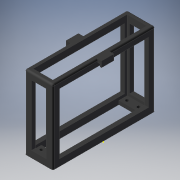
# Autodesk Inventor part: Battery Case2
Saved by Autodesk Inventor 2019 (Build 230136000, 136)
## iProperties
Created: 2019-01-06
Part Number: Battery Case2
Material: Generic
Document SubType Name: Modeling
Designer: Ashley
Density: 1 g/cm^3
Appearance: Default
Author: Ashley
Autodesk Inventor part; units mm, degrees
ref_plane "YZ Plane" through (0, 0, 0) normal (1, 0, 0) x (0, 1, 0)
ref_plane "XZ Plane" through (0, 0, 0) normal (0, 1, 0) x (-1, 0, 0)
ref_plane "XY Plane" through (0, 0, 0) normal (0, 0, 1) x (1, 0, 0)
sketch "Sketch1" plane through (0, 0, 0) normal (0, 1, 0) x (-1, 0, 0)
  point P0 (0, 0)
sketch "Sketch2" plane through (0, 0, 0) normal (0, 1, 0) x (-1, 0, 0)
  line L0 (34.7144, 60.4703) -> (0.7144, 60.4703)
  line L1 (0.7144, 60.4703) -> (0.7144, -63.8297)
  line L2 (0.7144, -63.8297) -> (34.7144, -63.8297)
  line L3 (34.7144, -63.8297) -> (34.7144, 60.4703)
  point P0 (0, 0)
  dimension "d0" = 124.3
  dimension "d1" = 34
  constraints: 8 end point, 2 parallel, 1 horizontal, 1 perpendicular
  measures "d0" distance of L2.end L0.start
  measures "d1" distance of L0.start L0.end
extrude "Extrusion1" add sketch "Sketch2" along normal blind 90
sketch "Sketch3" plane through (0, 90, 0) normal (0, 1, 0) x (1, 0, 0)
  line L0 (-34.7144, -60.4703) -> (-0.7144, -60.4703) construction
  line L1 (-0.7144, -60.4703) -> (-0.7144, 63.8297) construction
  line L2 (-0.7144, 63.8297) -> (-34.7144, 63.8297) construction
  line L3 (-34.7144, 63.8297) -> (-34.7144, -60.4703) construction
  line L4 (-29.7144, 58.8297) -> (-5.7144, 58.8297)
  line L5 (-5.7144, 58.8297) -> (-5.7144, -55.4703)
  line L6 (-5.7144, -55.4703) -> (-29.7144, -55.4703)
  line L7 (-29.7144, -55.4703) -> (-29.7144, 58.8297)
  point P0 (0, 0)
  dimension "d4" = 114.3
  dimension "d5" = 24
  dimension "d6" = 5
  dimension "d7" = 5
  dimension "d8" = 5
  dimension "d9" = 5
  constraints: 8 end point, 2 parallel, 1 horizontal, 1 perpendicular
  measures "d4" distance of L6.end L4.start
  measures "d5" distance of L5.end L6.end
  measures "d6" distance between parallel lines of L1 L5
  measures "d7" distance between parallel lines of L3 L7
  measures "d8" distance between parallel lines of L0 L6
  measures "d9" distance between parallel lines of L2 L4
extrude "Extrusion2" cut sketch "Sketch3" against normal blind 85.5
sketch "Sketch4" plane through (-0.7144, 0, 60.4703) normal (1, 0, 0) x (0, 0, -1)
  line L0 (124.3, 0) -> (124.3, 90) construction
  line L1 (0, 90) -> (124.3, 90) construction
  line L2 (54.65, 90) -> (69.65, 90)
  line L3 (69.65, 90) -> (69.65, 83)
  line L4 (69.65, 83) -> (54.65, 83)
  line L5 (54.65, 83) -> (54.65, 90)
  point P0 (60.4703, 0)
  dimension "d12" = 15
  dimension "d13" = 7
  dimension "d14" = 0
  dimension "d15" = 54.65
  constraints: 8 end point, 2 parallel, 1 horizontal, 1 perpendicular
  measures "d12" distance of L2.start L2.end
  measures "d13" distance of L2.end L3.end
  measures "d14" distance between parallel lines of L1 L2
  measures "d15" distance between parallel lines of L0 L3
extrude "Extrusion3" add sketch "Sketch4" along normal blind 4.5
sketch "Sketch5" plane through (-34.7144, 0, -63.8297) normal (-1, 0, 0) x (0, 0, 1)
  line L0 (124.3, 0) -> (124.3, 90) construction
  line L1 (0, 90) -> (124.3, 90) construction
  line L2 (54.65, 90) -> (69.65, 90)
  line L3 (69.65, 90) -> (69.65, 83)
  line L4 (69.65, 83) -> (54.65, 83)
  line L5 (54.65, 83) -> (54.65, 90)
  point P0 (63.8297, 0)
  dimension "d18" = 7
  dimension "d19" = 15
  dimension "d20" = 0
  dimension "d21" = 54.65
  constraints: 8 end point, 2 parallel, 1 horizontal, 1 perpendicular
  measures "d18" distance of L2.end L3.end
  measures "d19" distance of L3.end L4.end
  measures "d20" distance between parallel lines of L1 L2
  measures "d21" distance between parallel lines of L0 L3
extrude "Extrusion4" add sketch "Sketch5" along normal blind 4.5
sketch "Sketch6" plane through (-34.7144, 83, -9.1797) normal (0, -1, 0) x (1, 0, 0)
  line L0 (0, 15) -> (0, 0) construction
  line L1 (0, 15) -> (-4.5, 15) construction
  line L2 (-3, 0) -> (0, 0)
  line L3 (0, 0) -> (0, 15)
  line L4 (0, 15) -> (-3, 15)
  line L5 (-3, 15) -> (-3, 0)
  point P0 (34.7144, 9.1797)
  dimension "d24" = 15
  dimension "d25" = 3
  dimension "d26" = 0
  dimension "d27" = 0
  constraints: 8 end point, 2 parallel, 1 horizontal, 1 perpendicular
  measures "d24" distance of L4.end L2.start
  measures "d25" distance of L3.end L4.end
  measures "d26" distance between parallel lines of L0 L3
  measures "d27" distance between parallel lines of L1 L4
extrude "Extrusion5" cut sketch "Sketch6" against normal blind 3
sketch "Sketch7" plane through (-0.7144, 83, -9.1797) normal (0, -1, 0) x (1, 0, 0)
  line L0 (0, 0) -> (0, 15) construction
  line L1 (0, 15) -> (4.5, 15) construction
  line L2 (0, 15) -> (3, 15)
  line L3 (3, 15) -> (3, 0)
  line L4 (3, 0) -> (0, 0)
  line L5 (0, 0) -> (0, 15)
  point P0 (0.7144, 9.1797)
  dimension "d30" = 15
  dimension "d31" = 3
  dimension "d32" = 0
  dimension "d33" = 0
  constraints: 8 end point, 2 parallel, 1 horizontal, 1 perpendicular
  measures "d30" distance of L2.end L3.end
  measures "d31" distance of L2.start L2.end
  measures "d32" distance between parallel lines of L1 L2
  measures "d33" distance between parallel lines of L5 L0
extrude "Extrusion6" cut sketch "Sketch7" against normal blind 3
sketch "Sketch8" plane through (-34.7144, 0, 60.4703) normal (0, 0, 1) x (1, 0, 0)
  line L0 (0, 0) -> (34, 0) construction
  line L1 (34, 0) -> (34, 90) construction
  line L2 (0, 90) -> (34, 90) construction
  line L3 (0, 0) -> (0, 90) construction
  line L4 (8, 82) -> (26, 82)
  line L5 (26, 82) -> (26, 8)
  line L6 (26, 8) -> (8, 8)
  line L7 (8, 8) -> (8, 82)
  point P0 (34.7144, 0)
  dimension "d38" = 8
  dimension "d39" = 8
  dimension "d84" = 8
  dimension "d85" = 8
  constraints: 8 end point, 2 parallel, 1 horizontal, 1 perpendicular
  measures "d38" distance between parallel lines of L1 L5
  measures "d39" distance between parallel lines of L2 L4
  measures "d84" distance between parallel lines of L3 L7
  measures "d85" distance between parallel lines of L6 L0
extrude "Extrusion7" cut sketch "Sketch8" against normal blind 124.3
sketch "Sketch9" plane through (-0.7144, 0, 60.4703) normal (1, 0, 0) x (0, 0, -1)
  line L0 (0, 0) -> (0, 90) construction
  line L1 (0, 0) -> (124.3, 0) construction
  line L2 (124.3, 0) -> (124.3, 90) construction
  line L3 (69.65, 90) -> (124.3, 90) construction
  line L4 (8, 82) -> (116.3, 82)
  line L5 (116.3, 82) -> (116.3, 8)
  line L6 (116.3, 8) -> (8, 8)
  line L7 (8, 8) -> (8, 82)
  point P0 (60.4703, 0)
  dimension "d46" = 8
  dimension "d48" = 8
  dimension "d82" = 8
  dimension "d83" = 8
  constraints: 8 end point, 2 parallel, 1 horizontal, 1 perpendicular
  measures "d46" distance between parallel lines of L0 L7
  measures "d48" distance between parallel lines of L3 L4
  measures "d82" distance between parallel lines of L2 L5
  measures "d83" distance between parallel lines of L6 L1
extrude "Extrusion8" cut sketch "Sketch9" against normal blind 34
sketch "Sketch11" plane through (0, 0, 0) normal (0, -1, 0) x (1, 0, 0)
  line L0 (-34.7144, 60.4703) -> (-0.7144, 60.4703) construction
  line L1 (-34.7144, -63.8297) -> (-34.7144, 60.4703) construction
  line L2 (-0.7144, -63.8297) -> (-34.7144, -63.8297) construction
  line L3 (-0.7144, 60.4703) -> (-0.7144, -63.8297) construction
  circle A0 centre (-24.7144, -53.8297) radius 2.1
  circle A1 centre (-10.7144, -53.8297) radius 2.1
  circle A2 centre (-24.7144, 50.4703) radius 2.1
  circle A3 centre (-10.7144, 50.4703) radius 2.1
  line L4 (-29.7144, -48.8297) -> (-5.7144, -48.8297)
  line L5 (-5.7144, -48.8297) -> (-5.7144, 45.4703)
  line L6 (-5.7144, 45.4703) -> (-29.7144, 45.4703)
  line L7 (-29.7144, 45.4703) -> (-29.7144, -48.8297)
  point P0 (0, 0)
  dimension "d52" = 4.2
  dimension "d53" = 10
  dimension "d54" = 10
  dimension "d55" = 4.2
  dimension "d56" = 10
  dimension "d57" = 10
  dimension "d58" = 4.2
  dimension "d59" = 10
  dimension "d60" = 10
  dimension "d61" = 4.2
  dimension "d62" = 10
  dimension "d63" = 10
  dimension "d66" = 94.3
  dimension "d67" = 24
  dimension "d68" = 5
  dimension "d69" = 5
  dimension "d70" = 5
  dimension "d71" = 5
  constraints: 8 end point, 4 centre point, 2 parallel, 1 horizontal, 1 perpendicular
  measures "d52" diameter of A0
  measures "d53" distance from line of L2 A0.centre
  measures "d54" distance from line of L1 A0.centre
  measures "d55" diameter of A1
  measures "d56" distance from line of L2 A1.centre
  measures "d57" distance from line of L3 A1.centre
  measures "d58" diameter of A2
  measures "d59" distance from line of L0 A2.centre
  measures "d60" distance from line of L1 A2.centre
  measures "d61" diameter of A3
  measures "d62" distance from line of L0 A3.centre
  measures "d63" distance from line of L3 A3.centre
  measures "d66" distance of L6.end L4.start
  measures "d67" distance of L5.end L6.end
  measures "d68" distance from line of A2.centre L6
  measures "d69" distance from line of A0.centre L4
  measures "d70" distance between parallel lines of L1 L7
  measures "d71" distance between parallel lines of L3 L5
extrude "Extrusion9" cut sketch "Sketch11" against normal blind 5 contours A0 | A1 | A2 | A3
sketch "Sketch12" plane through (0, 0, 0) normal (0, -1, 0) x (1, 0, 0)
  circle A0 centre (-24.7144, 50.4703) radius 2.1 construction
  circle A1 centre (-24.7144, -53.8297) radius 2.1 construction
  line L0 (-34.7144, -63.8297) -> (-34.7144, 60.4703) construction
  line L1 (-0.7144, 60.4703) -> (-0.7144, -63.8297) construction
  line L2 (-29.7144, -48.8297) -> (-5.7144, -48.8297)
  line L3 (-5.7144, -48.8297) -> (-5.7144, 45.4703)
  line L4 (-5.7144, 45.4703) -> (-29.7144, 45.4703)
  line L5 (-29.7144, 45.4703) -> (-29.7144, -48.8297)
  point P0 (0, 0)
  dimension "d72" = 94.3
  dimension "d73" = 24
  dimension "d74" = 5
  dimension "d75" = 5
  dimension "d76" = 5
  dimension "d77" = 5
  constraints: 8 end point, 2 parallel, 1 horizontal, 1 perpendicular
  measures "d72" distance of L4.end L2.start
  measures "d73" distance of L3.end L4.end
  measures "d74" distance from line of A0.centre L4
  measures "d75" distance between parallel lines of L5 L0
  measures "d76" distance between parallel lines of L1 L3
  measures "d77" distance from line of A1.centre L2
extrude "Extrusion10" cut sketch "Sketch12" against normal blind 5
fillet "Fillet1" radius 2 10 edges at (-34.7144, 90, -36.5047) (-34.7144, 90, 33.1453) (-17.7144, 90, 60.4703) (-0.7144, 90, 33.1453) (-0.7144, 90, -36.5047) (-17.7144, 90, -63.8297) (-34.7144, 45, 60.4703) (-0.7144, 45, 60.4703) (-0.7144, 45, -63.8297) (-34.7144, 45, -63.8297)
equation "\"d38\" = d84"
equation "\"d39\" = d84"
equation "\"d85\" = d84"
equation "\"d48\" = d46"
equation "\"d82\" = d48"
equation "\"d83\" = d46"
equation "\"d52\" = d55"
equation "\"d55\" = d61"
equation "\"d58\" = d61"
body "Solid1"
